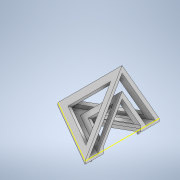
# Autodesk Inventor part: coltar5mmV2
Saved by Autodesk Inventor 2020 (Build 240168000, 168)
## iProperties
Created: 2022-02-13
Part Number: coltar5mmV2
Material: Generic
Document SubType Name: Modeling
Designer: Vlasciar
Density: 1 g/cm^3
Appearance: Default
Author: Vlasciar
Autodesk Inventor part; units mm, degrees
ref_plane "YZ Plane" through (0, 0, 0) normal (1, 0, 0) x (0, 1, 0)
ref_plane "XZ Plane" through (0, 0, 0) normal (0, 1, 0) x (-1, 0, 0)
ref_plane "XY Plane" through (0, 0, 0) normal (0, 0, 1) x (1, 0, 0)
sketch "Sketch1" plane through (0, 0, 0) normal (1, 0, 0) x (0, 1, 0)
  line L0 (0, 25) -> (0, -25)
  line L1 (0, -25) -> (43.3013, 0)
  line L2 (43.3013, 0) -> (0, 25)
  point P0 (0, 0)
  dimension "d0" = 50
  constraints: 6 end point, 2 equal length, 1 horizontal alignment, 1 midpoint, 1 vertical
  measures "d0" distance of L0.start L0.end
sketch "Sketch2" plane through (0, 0, 0) normal (0, 1, 0) x (-1, 0, 0)
  line L0 (0, 25) -> (43.3013, 0)
  line L1 (43.3013, 0) -> (0, -25)
  line L2 (0, -25) -> (0, 25)
  point P0 (0, 0)
  point P1 (0, 0)
  dimension "d1" = 50
  constraints: 6 end point, 2 equal length, 1 coincident, 1 horizontal alignment, 1 midpoint, 1 vertical
  measures "d1" distance of L0.start L0.end
extrude "Extrusion1" add sketch "Sketch2" against normal blind 2
sketch "Sketch3" plane through (0, 0, 0) normal (0, 1, 0) x (1, 0, 0)
  line L0 (-43.3013, 0) -> (0, -25) projected
  line L1 (0, -25) -> (0, 25) projected
  line L2 (0, 25) -> (-43.3013, 0) projected
  point P0 (0, 0)
ref_plane "Work Plane1" through (0, 43.3013, 0) normal (-0.4472136, 0.4472136, 0.7745967) x (0, -0.8660254, 0.5)
ref_plane "Work Plane2" through (0, 0, -25) normal (0.4472136, -0.4472136, 0.7745967) x (0, 0.8660254, 0.5)
extrude "Extrusion2" add sketch "Sketch1" against normal up to surface surface through (0, 43.3013, 0) normal (-0.4472136, 0.4472136, 0.7745967)
split "Split1" plane through (0, 0, -25) removes the side toward (-0.4472136, 0.4472136, -0.7745967)
shell "Shell1" thickness 2 removed faces 1 at (0, 14.4338, 0)
sketch "Sketch4" plane through (0, -2, 25) normal (1, 0, 0) x (0, 0, -1)
  line L0 (47.418, 2) -> (2.582, 2) projected
  line L1 (2.582, 2) -> (25, 40.8291) projected
  line L2 (25, 40.8291) -> (47.418, 2) projected
  line L3 (25, 40.8291) -> (25, 2) projected
  line L4 (25, 30.3291) -> (8.6442, 2)
  line L5 (25, 30.3291) -> (41.3558, 2)
  dimension "d7" = 5.25
  constraints: 4 end point, 3 point on line, 2 parallel
  measures "d7" distance between parallel lines of L2 L5
sketch "Sketch5" plane through (0, 0, 22.418) normal (0, 1, 0) x (1, 0, 0)
  line L0 (-38.8291, 22.418) -> (0, 0) projected
  line L1 (0, 44.836) -> (0, 0) projected
  line L2 (0, 44.836) -> (-38.8291, 22.418) projected
  line L3 (0, 47.418) -> (0, -2.582) projected
  line L4 (0, 6.0622) -> (-28.3291, 22.418)
  line L5 (-28.3291, 22.418) -> (0, 38.7738)
  point P0 (0, 22.418)
  dimension "d8" = 5.25
  dimension "d9" = 5.25
  constraints: 4 end point, 2 parallel, 2 point on line
  measures "d8" distance between parallel lines of L0 L4
  measures "d9" distance between parallel lines of L2 L5
ref_plane "Work Plane3" through (0, 28.3291, 0) normal (0.4472136, -0.4472136, -0.7745967) x (0, -0.8660254, 0.5)
ref_plane "Work Plane4" through (0, 28.3291, 0) normal (0.4472136, -0.4472136, 0.7745967) x (0, -0.8660254, -0.5)
extrude "Extrusion3" add sketch "Sketch4" along normal up to surface separate body contours L0 L3 L5 | L0 L4 L3 surface through (0, 28.3291, 0) normal (0.4472136, -0.4472136, -0.7745967)
split "Split2" plane through (0, 28.3291, 0) removes the side toward (-0.4472136, 0.4472136, -0.7745967) bodies 2
shell "Shell2" thickness 2 removed faces 1 at (0, 9.443, 0) bodies 2
sketch "Sketch6" plane through (-43.3013, 0, 0) normal (-0.4472136, 0.4472136, 0.7745967) x (0.5477226, -0.5477226, 0.6324555)
  line L0 (0, 61.2372) -> (0, 0) projected
  line L1 (0, 0) -> (39.5285, 30.6186) projected
  line L2 (0, 61.2372) -> (39.5285, 30.6186) projected
  line L3 (5, 10.1975) -> (5, 51.0397)
  line L4 (5, 51.0397) -> (31.3635, 30.6186)
  line L5 (31.3635, 30.6186) -> (5, 10.1975)
  point P0 (23.7171, 30.6186)
  dimension "d13" = 5
  dimension "d14" = 5
  dimension "d15" = 5
  constraints: 6 end point, 3 parallel
  measures "d13" distance between parallel lines of L0 L3
  measures "d14" distance between parallel lines of L2 L4
  measures "d15" distance between parallel lines of L5 L1
extrude "Extrusion4" cut sketch "Sketch6" against normal blind 2 contours L3 L4 L5 bodies 1
sketch "Sketch7" plane through (-43.3013, 0, 0) normal (-0.4472136, 0.4472136, -0.7745967) x (-0.5477226, 0.5477226, 0.6324555)
  line L0 (-39.5285, 30.6186) -> (0, 0) projected
  line L1 (0, 61.2372) -> (0, 0) projected
  line L2 (-39.5285, 30.6186) -> (0, 61.2372) projected
  line L3 (-5, 51.0397) -> (-5, 10.1975)
  line L4 (-5, 10.1975) -> (-31.3635, 30.6186)
  line L5 (-31.3635, 30.6186) -> (-5, 51.0397)
  point P0 (-23.7171, 30.6186)
  dimension "d18" = 5
  dimension "d19" = 5
  dimension "d20" = 5
  constraints: 6 end point, 3 parallel
  measures "d18" distance between parallel lines of L2 L5
  measures "d19" distance between parallel lines of L1 L3
  measures "d20" distance between parallel lines of L0 L4
extrude "Extrusion5" cut sketch "Sketch7" against normal blind 2 contours L3 L4 L5 bodies 1
sketch "Sketch8" plane through (-28.3291, 0, 0) normal (-0.4472136, 0.4472136, -0.7745967) x (-0.5477226, 0.5477226, 0.6324555)
  line L0 (0, 0) -> (-25.8608, 20.0317) projected
  line L1 (0, 40.0634) -> (0, 0) projected
  line L2 (-25.8608, 20.0317) -> (0, 40.0634) projected
  line L3 (-4, 31.9054) -> (-4, 8.158)
  line L4 (-4, 8.158) -> (-19.3289, 20.0317)
  line L5 (-19.3289, 20.0317) -> (-4, 31.9054)
  point P0 (-15.5165, 20.0317)
  dimension "d23" = 4
  dimension "d24" = 4
  dimension "d25" = 4
  constraints: 6 end point, 3 parallel
  measures "d23" distance between parallel lines of L0 L4
  measures "d24" distance between parallel lines of L1 L3
  measures "d25" distance between parallel lines of L2 L5
extrude "Extrusion6" cut sketch "Sketch8" against normal blind 2 contours L3 L4 L5 bodies 2
sketch "Sketch9" plane through (-28.3291, 0, 0) normal (-0.4472136, 0.4472136, 0.7745967) x (0.5477226, -0.5477226, 0.6324555)
  line L0 (0, 40.0634) -> (0, 0) projected
  line L1 (0, 0) -> (25.8608, 20.0317) projected
  line L2 (25.8608, 20.0317) -> (0, 40.0634) projected
  line L3 (4, 8.158) -> (19.3289, 20.0317)
  line L4 (19.3289, 20.0317) -> (4, 31.9054)
  line L5 (4, 31.9054) -> (4, 8.158)
  point P0 (15.5165, 20.0317)
  dimension "d28" = 4
  dimension "d29" = 4
  dimension "d30" = 4
  constraints: 6 end point, 3 parallel
  measures "d28" distance between parallel lines of L0 L5
  measures "d29" distance between parallel lines of L1 L3
  measures "d30" distance between parallel lines of L2 L4
extrude "Extrusion7" cut sketch "Sketch9" against normal blind 2 contours L5 L4 L3 bodies 2
sketch "Sketch10" plane through (0, 2, 12.6191) normal (0, 1, 0) x (1, 0, 0)
  line L0 (-21.857, 12.6191) -> (0, 25.2383) projected
  line L1 (-21.857, 12.6191) -> (0, 0) projected
  line L2 (0, 25.2383) -> (0, 0) projected
  point P0 (0, 12.6191)
extrude "Extrusion8" cut sketch "Sketch10" against normal blind 6 bodies 2 1
sketch "Sketch11" plane through (0, -2, 0) normal (0, -1, 0) x (1, 0, 0)
  line L0 (0, 0) -> (-38.8291, 0) projected
  circle A0 centre (-30.914, 0) radius 0.625
  circle A1 centre (-5.1819, -16.0247) radius 0.625
  circle A2 centre (-5.1819, 16.0247) radius 0.625
  dimension "d35" = 1.25
  dimension "d36" = 1.25
  dimension "d37" = 1.25
  constraints: 3 centre point, 1 point on line
  measures "d35" diameter of A0
  measures "d36" diameter of A1
  measures "d37" diameter of A2
extrude "Extrusion9" add sketch "Sketch11" along normal blind 5 bodies 1
draft "FaceDraft1" angle 10 pull direction (0, -1, 0) faces at (-4.565, -5.3333, 15.9244) (-4.565, -5.3333, -16.1249) (-30.2971, -5.3333, -0.1003) fixed edges at (-5.8069, -7, 16.0247) (-5.8069, -7, -16.0247) (-31.539, -7, 0)
body "Solid1"
body "Solid2"
